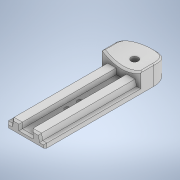
# Autodesk Inventor part: Union_Telescopio
Saved by Autodesk Inventor 2021 (Build 250183000, 183)
## iProperties
Created: 2021-01-10
Part Number: Union_Telescopio
Material: Generic
Document SubType Name: Modeling
Designer: jorge
Density: 1 g/cm^3
Appearance: Default
Author: jorge
Autodesk Inventor part; units mm, degrees
ref_plane "YZ Plane" through (0, 0, 0) normal (1, 0, 0) x (0, 1, 0)
ref_plane "XZ Plane" through (0, 0, 0) normal (0, 1, 0) x (-1, 0, 0)
ref_plane "XY Plane" through (0, 0, 0) normal (0, 0, 1) x (1, 0, 0)
sketch "Sketch1" plane through (0, 0, 0) normal (0, 1, 0) x (-1, 0, 0)
  line L0 (0, 0) -> (-43.5, 0)
  line L1 (-43.5, 0) -> (-43.5, -108)
  line L2 (-43.5, -108) -> (0, -108)
  line L3 (0, -108) -> (0, 0)
  circle A0 centre (-21.75, -47) radius 3
  circle A1 centre (-21.75, -61) radius 3
  dimension "d0" = 43.5
  dimension "d1" = 108
  dimension "d2" = 6
  dimension "d3" = 6
  dimension "d4" = 21.75
  dimension "d5" = 21.75
  dimension "d6" = 47
  dimension "d7" = 47
  constraints: 8 end point, 2 centre point, 2 parallel, 1 horizontal, 1 perpendicular
  measures "d0" distance of L2.end L1.end
  measures "d1" distance of L1.end L0.end
  measures "d2" diameter of A0
  measures "d3" diameter of A1
  measures "d4" distance from line of A0.centre L3
  measures "d5" distance from line of A1.centre L3
  measures "d6" distance from line of A0.centre L0
  measures "d7" distance from line of A1.centre L2
extrude "Extrusion1" add sketch "Sketch1" along normal blind 5
sketch "Sketch2" plane through (0, 5, 0) normal (0, 1, 0) x (1, 0, 0)
  line L0 (0, 0) -> (43.5, 0) projected
  line L1 (43.5, 108) -> (0, 108) projected
  line L2 (15.75, 0) -> (27.75, 0)
  line L3 (27.75, 0) -> (27.75, 108)
  line L4 (27.75, 108) -> (15.75, 108)
  line L5 (15.75, 108) -> (15.75, 0)
  circle A0 centre (21.75, 61) radius 3 projected
  line L6 (15.75, 0) -> (6.25, 0)
  line L7 (6.25, 0) -> (6.25, 108)
  line L8 (6.25, 108) -> (15.75, 108)
  line L9 (15.75, 108) -> (15.75, 0)
  line L10 (27.75, 0) -> (37.25, 0)
  line L11 (37.25, 0) -> (37.25, 108)
  line L12 (37.25, 108) -> (27.75, 108)
  line L13 (27.75, 108) -> (27.75, 0)
  dimension "d10" = 12
  dimension "d11" = 6
  dimension "d12" = 9.5
  dimension "d13" = 9.5
  constraints: 24 end point, 6 parallel, 4 point on line, 3 horizontal, 3 perpendicular
  measures "d10" distance between parallel lines of L3 L5
  measures "d11" distance from line of A0.centre L5
  measures "d12" distance between parallel lines of L5 L7
  measures "d13" distance between parallel lines of L11 L3
extrude "Extrusion2" add sketch "Sketch2" along normal blind 6.5 contours L7 L1 L5 L0 | L3 L1 L11 L0
sketch "Sketch3" plane through (43.5, 0, -108) normal (0, 0, -1) x (-1, 0, 0)
  line L0 (27.75, 11.5) -> (37.25, 11.5) projected
  line L1 (37.25, 5) -> (37.25, 11.5) projected
  line L2 (37.25, 11.5) -> (37.25, 5)
  line L3 (37.25, 5) -> (38.75, 5)
  line L4 (37.25, 5) -> (43.5, 5) projected
  line L5 (38.75, 5) -> (37.25, 11.5)
  line L6 (6.25, 11.5) -> (15.75, 11.5) projected
  line L7 (6.25, 11.5) -> (6.25, 4.9469)
  line L8 (6.25, 5) -> (6.25, 11.5) projected
  line L9 (0, 5) -> (6.25, 5) projected
  line L10 (6.25, 11.5) -> (6.25, 5)
  line L11 (6.25, 5) -> (4.75, 5)
  line L12 (4.75, 5) -> (6.25, 11.5)
  point P0 (43.5, 0)
  point P1 (4.75, 5)
  dimension "d16" = 1.5
  dimension "d17" = 1.5
  constraints: 14 end point, 2 vertical, 1 collinear, 1 perpendicular, 1 point on line
  measures "d16" distance of L1.start L3.end
  measures "d17" distance of L8.start L11.end
extrude "Extrusion3" add sketch "Sketch3" against normal up to surface (108 mm away)
sketch "Sketch4" plane through (0, 0, 0) normal (0, -1, 0) x (1, 0, 0)
  line L0 (43.5, 0) -> (43.5, -108) projected
  line L1 (43.5, -108) -> (0, -108)
  line L2 (0, -108) -> (0, -123)
  line L3 (0, -123) -> (43.5, -123)
  line L4 (43.5, -123) -> (43.5, -108)
  line L5 (0, -108) -> (0, 0) projected
  arc A0 (0, -123) -> (43.5, -123) centre (21.75, -123) ccw
  dimension "d20" = 15
  constraints: 8 end point, 2 parallel, 2 point on circle, 2 tangent, 1 centre point, 1 collinear, 1 horizontal, 1 perpendicular
  measures "d20" distance between parallel lines of L3 L1
extrude "Extrusion4" add sketch "Sketch4" against normal blind 15.5
sketch "Sketch12" plane through (0, 15.5, -108) normal (0, 0, 1) x (1, 0, 0)
  arc A0 (0, 7.1881) -> (43.5, 7.1881) centre (21.75, 36.5) ccw
  line L0 (0, -10.5) -> (0, 0) projected
  line L1 (0, 0) -> (0, 7.1881)
  line L2 (0, 0) -> (43.5, 0) projected
  line L3 (43.5, 0) -> (43.5, 7.1881)
  line L4 (43.5, 0) -> (0, 0)
  line L5 (43.5, -10.5) -> (43.5, 0) projected
  line L6 (0, 7.1881) -> (43.5, 7.1881)
  point P0 (0, -15.5)
  point P1 (21.75, 0)
  point P2 (21.75, 0)
  dimension "d48" = 36.5
  constraints: 8 end point, 3 point on circle, 2 collinear, 1 centre point, 1 midpoint, 1 parallel, 1 perpendicular
  measures "d48" radius of A0
extrude "Extrusion11" add sketch "Sketch12" against normal up to surface contours A0 L2 L1 | A0 L3 L2 round surface about axis through (21.75, 0, -123) along (0, 1, 0) radius 21.75 far side no
sketch "Sketch13" plane through (0, 0, 0) normal (0, -1, 0) x (1, 0, 0)
  arc A0 (0, -123) -> (43.5, -123) centre (21.75, -123) ccw projected
  circle A1 centre (21.75, -123) radius 4.05
  point P0 (0, 0)
  dimension "d51" = 8.1
  constraints: 1 centre point, 1 coincident
  measures "d51" diameter of A1
extrude "Extrusion12" cut sketch "Sketch13" against normal up to surface round surface about axis through (21.75, 52, -108) along (0, 0, -1) radius 36.5 far side no
chamfer "Chamfer2" distance 2 angle 45 16 edges at (21.75, 15.5, -108) (43.5, 22.6881, -115.5) (38.2818, 19.4585, -137.1337) (5.2182, 19.4585, -137.1337) (0, 22.6881, -115.5) (0, 2.5, 0) (2.375, 5, 0) (5.5, 8.25, 0) (11, 11.5, 0) (15.75, 8.25, 0) (21.75, 5, 0) (27.75, 8.25, 0) (32.5, 11.5, 0) (38, 8.25, 0) (43.5, 2.5, 0) (41.125, 5, 0)
body "Solid1"
